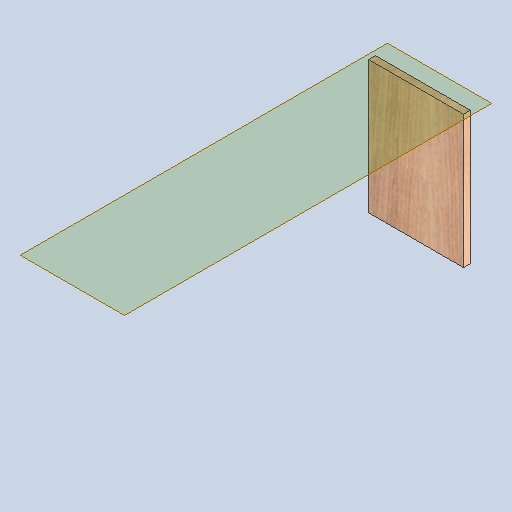
# Autodesk Inventor part: Deska_bocni
Saved by Autodesk Inventor 2024.2 (Build 282272000, 272)
## iProperties
Created: 2024-03-09
Part Number: Deska_bocni
Material: Dřevo (Bříza)
Document SubType Name: Modeling
Designer: lukyv
Density: 0.55 g/cm^3
Appearance: Bříza – přírodní leštěná
Author: lukyv
Autodesk Inventor part; units mm, degrees
ref_plane "YZ Plane" through (0, 0, 0) normal (1, 0, 0) x (0, 1, 0)
ref_plane "XZ Plane" through (0, 0, 0) normal (0, 1, 0) x (-1, 0, 0)
ref_plane "XY Plane" through (0, 0, 0) normal (0, 0, 1) x (1, 0, 0)
ref_plane "Pracovní rovina1" through (0, 0, -12) normal (0, 0, -1) x (-1, 0, 0)
sketch "Náčrt1" plane through (0, 0, -12) normal (0, 0, -1) x (-1, 0, 0)
  line L0 (-125, 440) -> (-125, 40) projected
  line L1 (-125, 40) -> (125, 40) projected
  line L2 (125, 40) -> (125, 440) projected
  line L3 (125, 440) -> (-125, 440) projected
  line L4 (-125, 440) -> (-125, 40) projected
  line L5 (-125, 40) -> (125, 40) projected
  line L6 (125, 40) -> (125, 440) projected
  line L7 (125, 440) -> (-125, 440) projected
  line L8 (125, 440) -> (-125, 440)
  line L9 (-125, 440) -> (-125, 422)
  line L10 (-125, 422) -> (125, 422)
  line L11 (125, 422) -> (125, 440)
  point P0 (0, 0)
  dimension "d0" = 18
  constraints: 8 end point, 2 parallel, 1 horizontal, 1 perpendicular, 1 point on line
  measures "d0" distance of L9.end L8.end
extrude "Vysunutí1" add sketch "Náčrt1" along normal blind 350 contours L3 L2 L10 L0
